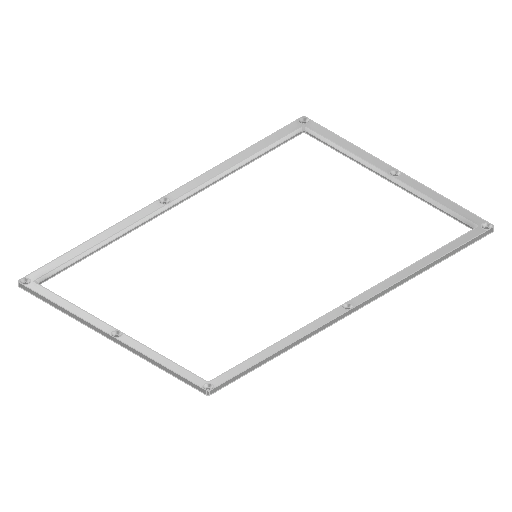
# Autodesk Inventor part: 3DP_PLA_Front_Mounting_Bracket
Saved by Autodesk Inventor 2026.1 (Build 301233000, 233)
## iProperties
Created: 2024-09-01
Part Number: 3DP_PLA_Front_Mounting_Bracket
Material: Generic
Document SubType Name: Modeling
Designer: User
Density: 1 g/cm^3
Appearance: Rubber - Black - Version 1.1
Author: User
Autodesk Inventor part; units mm, degrees
ref_plane "YZ Plane" through (0, 0, 0) normal (1, 0, 0) x (0, 1, 0)
ref_plane "XZ Plane" through (0, 0, 0) normal (0, 1, 0) x (-1, 0, 0)
ref_plane "XY Plane" through (0, 0, 0) normal (0, 0, 1) x (1, 0, 0)
sketch "Sketch1" plane through (0, 0, 0) normal (0, 1, 0) x (-1, 0, 0)
  line L0 (71, 106.5) -> (-71, 106.5)
  line L1 (-71, 106.5) -> (-71, -106.5)
  line L2 (-71, -106.5) -> (71, -106.5)
  line L3 (71, -106.5) -> (71, 106.5)
  line L4 (64.5, 100) -> (-64.5, 100)
  line L5 (-64.5, 100) -> (-64.5, -100)
  line L6 (-64.5, -100) -> (64.5, -100)
  line L7 (64.5, -100) -> (64.5, 100)
  line L8 (63.5, 99) -> (-63.5, 99)
  line L9 (-63.5, 99) -> (-63.5, -99)
  line L10 (-63.5, -99) -> (63.5, -99)
  line L11 (63.5, -99) -> (63.5, 99)
  line L12 (68, 103.5) -> (-68, 103.5)
  line L13 (-68, 103.5) -> (-68, -103.5)
  line L14 (-68, -103.5) -> (68, -103.5)
  line L15 (68, -103.5) -> (68, 103.5)
  point P0 (0, 0)
  point P1 (68, 0)
  point P2 (0, -103.5)
  point P3 (-68, 0)
  point P4 (0, 103.5)
  dimension "d0" = 142
  dimension "d1" = 213
  dimension "d2" = 71
  dimension "d3" = 106.5
  dimension "d4" = 129
  dimension "d5" = 200
  dimension "d6" = 64.5
  dimension "d7" = 100
  dimension "d8" = 1
  dimension "d22" = 3
  constraints: 32 end point, 8 parallel, 4 coincident, 4 midpoint, 4 perpendicular, 2 horizontal, 6 other
  measures "d0" distance of L2.end L1.end
  measures "d1" distance of L1.end L0.end
  measures "d2" distance from line of L3 point (0, 0)
  measures "d3" distance from line of L2 point (0, 0)
  measures "d4" distance of L6.end L5.end
  measures "d5" distance of L5.end L4.end
  measures "d6" distance from line of point (0, 0) L7
  measures "d7" distance from line of L4 point (0, 0)
  measures "d8" distance between parallel lines of L7 L11
  measures "d22" distance between parallel lines of L3 L15
extrude "Extrusion1" add sketch "Sketch1" along normal blind 3 contours L3 L2 L1 L0 | L7 L6 L5 L4 | L15 L14 L13 L12
hole "Hole1" at (0, 0, 103.5) at (-68, 0, 103.5) at (-68, 0, 0) at (-68, 0, -103.5) at (0, 0, -103.5) at (68, 0, -103.5) at (68, 0, 0) at (68, 0, 103.5) direction (0, 1, 0) diameter 3.1 end through all
chamfer "Chamfer1" distance 1.5 angle 45 4 edges at (-63.5, 3, 0) (0, 3, 99) (63.5, 3, 0) (0, 3, -99)
chamfer "Chamfer2" distance 1.5 angle 45 8 edges at (-68, 3, 1.55) (-68, 3, -101.95) (-68, 3, 105.05) (68, 3, 105.05) (68, 3, 1.55) (68, 3, -101.95) (0, 3, -101.95) (0, 3, 105.05)
fillet "Fillet1" radius 1 12 edges at (-71, 1.5, 106.5) (71, 1.5, 106.5) (71, 1.5, -106.5) (-71, 1.5, -106.5) (-63.5, 0.75, -99) (-64.25, 2.25, -99.75) (63.5, 0.75, -99) (64.25, 2.25, -99.75) (63.5, 0.75, 99) (64.25, 2.25, 99.75) (-64.25, 2.25, 99.75) (-63.5, 0.75, 99)
equation "\"d2\" = 0.5 * d0"
equation "\"d3\" = 0.5 * d1"
equation "\"d6\" = 0.5 * d4"
equation "\"d7\" = 0.5 * d5"
body "Solid1"
